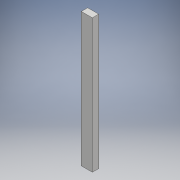
# Autodesk Inventor part: PL_rod_duoble
Saved by Autodesk Inventor 2018.3 (Build 223284000, 284)
## iProperties
Created: 2020-08-29
Part Number: PL_rod_duoble
Material: Generic
Document SubType Name: Modeling
Designer: chris
Density: 1 g/cm^3
Appearance: Default
Author: chris
Autodesk Inventor part; units mm, degrees
ref_plane "YZ Plane" through (0, 0, 0) normal (1, 0, 0) x (0, 1, 0)
ref_plane "XZ Plane" through (0, 0, 0) normal (0, 1, 0) x (-1, 0, 0)
ref_plane "XY Plane" through (0, 0, 0) normal (0, 0, 1) x (1, 0, 0)
sketch "Sketch1" plane through (0, 0, 0) normal (0, 0, 1) x (1, 0, 0)
  line L0 (-14, -7.9) -> (14, -7.9)
  line L1 (14, -7.9) -> (14, 8.3)
  line L2 (14, 8.3) -> (-14, 8.3)
  line L3 (-14, 8.3) -> (-14, -7.9)
  line L4 (-13, 7.3) -> (13, 7.3)
  line L5 (13, 7.3) -> (13, -6.9)
  line L6 (13, -6.9) -> (-13, -6.9)
  line L7 (-13, -6.9) -> (-13, 7.3)
  dimension "d2" = 1
  constraints: 16 end point, 4 parallel, 2 perpendicular, 2 vertical, 1 horizontal, 3 other
  measures "d2" distance between parallel lines of L2 L4
extrude "Extrusion1" add sketch "Sketch1" along normal blind 340
sketch "Sketch2" plane through (0, 0, 340) normal (0, 0, 1) x (1, 0, 0)
  line L0 (14, 8.3) -> (-14, 8.3) construction
  line L1 (14, -7.9) -> (14, 8.3) construction
  line L2 (-14, 8.3) -> (14, 8.3)
  line L3 (14, 8.3) -> (14, -7.9)
  line L4 (14, -7.9) -> (-14, -7.9)
  line L5 (-14, -7.9) -> (-14, 8.3)
  point P0 (0, 0)
  constraints: 8 end point, 2 parallel, 1 horizontal, 1 perpendicular
extrude "Extrusion2" add sketch "Sketch2" against normal blind 2
sketch "Sketch3" plane through (0, 0, 0) normal (0, 0, -1) x (-1, 0, 0)
  line L0 (14, -7.9) -> (-14, -7.9) construction
  line L1 (14, -7.9) -> (-14, -7.9)
  line L2 (-14, -7.9) -> (-14, 8.3)
  line L3 (-14, 8.3) -> (14, 8.3)
  line L4 (14, 8.3) -> (14, -7.9)
  point P0 (0, 0)
  constraints: 8 end point, 2 parallel, 1 horizontal, 1 perpendicular
extrude "Extrusion3" add sketch "Sketch3" against normal blind 2
body "Solid1"
